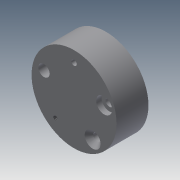
# Autodesk Inventor part: Part2
Saved by Autodesk Inventor 2015 (Build 190159000, 159)
## iProperties
Created: 2016-11-08
Part Number: Part2
Material: Generic
Document SubType Name: Modeling
Designer: Aniket Pant
Density: 1 g/cm^3
Appearance: Default
Author: Aniket Pant
Autodesk Inventor part; units mm, degrees
ref_plane "YZ Plane" through (0, 0, 0) normal (1, 0, 0) x (0, 1, 0)
ref_plane "XZ Plane" through (0, 0, 0) normal (0, 1, 0) x (-1, 0, 0)
ref_plane "XY Plane" through (0, 0, 0) normal (0, 0, 1) x (1, 0, 0)
sketch "Sketch1" plane through (0, 0, 0) normal (0, 0, 1) x (1, 0, 0)
  circle A0 centre (0, 0) radius 50.8
  dimension "d0" = 101.6
  constraints: 1 centre point, 1 coincident
  measures "d0" diameter of A0
extrude "Extrusion1" add sketch "Sketch1" along normal blind 38.1
sketch "Sketch2" plane through (0, 0, 38.1) normal (0, 0, 1) x (1, 0, 0)
  circle A0 centre (0, 0) radius 50.8 projected
  point P0 (0, 37.809)
  point P1 (-35.9585, 11.6836)
  point P2 (-22.2236, -30.5881)
  point P3 (22.2236, -30.5881)
  point P4 (35.9585, 11.6836)
  dimension "d5" = 360
  constraints: 6 other
hole "Hole1" at (0, 37.809, 38.1) direction (0, 0, -1) diameter 6.35 end through all
hole "Hole2" at (35.9585, 11.6836, 38.1) direction (0, 0, -1) diameter 9.525 end through all counterbore diameter 19.05 counterbore depth 6.35
hole "Hole3" at (22.2236, -30.5881, 38.1) direction (0, 0, -1) diameter 9.525 end through all countersink diameter 19.05 countersink angle 82
hole "Hole4" at (-22.2236, -30.5881, 38.1) direction (0, 0, -1) diameter 4.9784 end through all thread size "1/4-20 UNC" class "1B" standard "ANSI Unified Screw Threads"
hole "Hole5" at (-35.9585, 11.6836, 38.1) direction (0, 0, -1) diameter 13.4874 end through all clearance for "Hex Head Bolt" size "1/2" standard "Ansi Unified Screw Threads"
body "Solid1"
